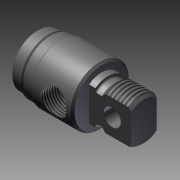
# Autodesk Inventor part: 04P0000_rear_head
Saved by Autodesk Inventor 2011 SP1 (Build 150282100, 282)
## iProperties
Created: 2015-01-23
Part Number: 04P0000_rear_head
Catalog Web Link: www.cadenas.de
Description: Rear Head-Original Line - Standard Air Cylinders
Vendor: BIMBA
Document SubType Name: Modeling
Designer: psAdmin
Manufacturer: BIMBA
Mass: 8.73981 g
Surface Area: 40.5299 cm^2
Volume: 8.73981 cm^3
Density: 1 g/cm^3
Category: PARTsolutions
Company: BIMBA
Title: 04P0000_rear_head
Author: Cadenas PARTsolutions
Comments: Original Line - Standard Air Cylinders
PSOL_IDENT_0: {$CADENAS_DATA\23d-libs\bimba\bimba\bimba_imperial\bimba_full_line\original_line_cylinders\standard_
PSOL_IDENT_1: air_cylinders\rear_head.prj},229 {VTYP=3D},{NB=04P0000_rear_head},{LINA=04P0000_rear_head},{NN=Rear
PSOL_IDENT_2: Head},{DATE=30.06.2014 06:34:23},{GEOMDATE=30.06.2014 06:34:00},{VERSION=},{LINEID=40},{LINESUBID=-1
PSOL_IDENT_3: },{WBVAR=MNT,ACTING,DER,Q,T1,T2,T3,T4,TRIM,Y,K,MB,CUSH,FBON}  {NB=04P0000_rear_head},{LINA=04P0000_r
PSOL_IDENT_4: ear_head},{KT=DUMMY},{PN=04P0000},{BORE=0.75000},{BOREPN=04},{MNT=P},{MNTALG='' , 'Front Nose' , 'P'
PSOL_IDENT_5: , 'Rear Pivot' , 'LS' , 'Built-in Valve LS' , 'DX' , 'Double End' , 'BR' , 'Rear Block' , 'BRT' , '
PSOL_IDENT_6: Rear Trunnion' , 'A' , 'Adjustable Stroke'},{ACTING=},{ACTINGALG= '' , 'Single Acting' , 'R' , 'Reve
PSOL_IDENT_7: rse/Double Acting'   },{DER=},{DERALG= '' , 'Standard' },{Q=},{T1=},{T2=},{T3=},{T4=},{TRIM=0},{Y=},
PSOL_IDENT_8: {K=},{KALG= '', 'without K', 'K', 'with K' },{MB=0},{A1=1.5940},{A1N=0.5310},{A1P=1.5940},{A1B=1.094
PSOL_IDENT_9: 0},{A1S=1.2190},{A2=0.219},{A2N=0.2190},{A3=0.0300},{D1=0.8625},{D1N=0.8050},{D1P=0.8625},{D1B=0.832
PSOL_IDENT_10: 5},{D2=0.7615},{C1=0.0300},{C2=0.0000},{NDM=0.4050},{TAB=NPT},{NDMDP=0.3020},{D3=0.3440},{A4=0.1880}
PSOL_IDENT_11: ,{A5=0.6200},{D4=0.0000},{A6=0.0000},{A7=0.7500},{A8=0.1250},{D5=0.8170},{D6=0.3120},{A9=0.8440},{ND
PSOL_IDENT_12: M2=0.6250},{TAB2=UNF},{C11=0.0300},{C22=0.0000},{C33=0.0227},{C44=0.0300},{A10=0.3725},{A11=0.0000},
PSOL_IDENT_13: {NDM3=0.4050},{NDM3N=0.4050},{NDM3B=0.4050},{TAB3=NPT},{TAB3N=NPT},{TAB3B=NPT},{A12=0.688},{A12N=0.6
PSOL_IDENT_14: 880},{A12B=0.6560},{A13=1.3120},{D7=0.2520},{D8=0.6225},{A14=0.0940},{A15=0.0855},{D9=0.5385},{R1=0.
PSOL_IDENT_15: 0350},{X1=0.0000},{X2=0.0000},{CX=0.0000},{CC=0.0000},{CON=1},{S1=1.0000},{DB=0.2500},{X1B=0.4380},{
PSOL_IDENT_16: X2B=0.0310},{A8B=0.1250},{A9B=0.8750},{MODEL=1},{NDM4=0.1900},{TAB4=UNF},{NDM4DP=0.2500},{BC=1.0000}
PSOL_IDENT_17: ,{B1=0.7150},{B2=0.5000},{B3=0.5000},{ON=0},{ON2=1},{G1=0.1250},{G2=0.5620},{G3=0.6250},{G4=0.6250},
PSOL_IDENT_18: {GD=0.2520},{G5=0.6250},{G6=0.3725},{RON=0},{H1=1.1175},{H2=0.8170},{H3=0.1250},{H4=0.0350},{H5=0.94
PSOL_IDENT_19: 20},{H6=0.5620},{F=0.4380},{PNUT=1.0630},{CUSH=0},{CC11=0.238},{CC111=0.2380},{CC22=0.2750},{CC33=0.
PSOL_IDENT_20: 1950},{CC44=0.3700},{CC55=0.5350},{CD1=0.1900},{CD2=0.1500},{CD3=0.0725},{CNDM3=0.1380},{CTAB3=UNF},
PSOL_IDENT_21: {OLEN=1.3120},{OD=0.3455},{STDIS=0.1560},{STDIS1=0.1560},{BUSHCON=D-3543},{BUSHL=0.3700},{FBON=0},{L
PSOL_IDENT_22: CD=0.0000}
SUPPLIER: BIMBA
ARTICLENO: 04P0000_rear_head
BOMINFO: 04P0000_rear_head
CREATOR: CADENAS GmbH
Autodesk Inventor part; units mm, degrees
ref_plane "YZ Plane" through (0, 0, 0) normal (1, 0, 0) x (0, 1, 0)
ref_plane "XZ Plane" through (0, 0, 0) normal (0, 1, 0) x (-1, 0, 0)
ref_plane "XY Plane" through (0, 0, 0) normal (0, 0, 1) x (1, 0, 0)
sketch "Sketch_8" plane through (0, 0, 0) normal (0, 0, 1) x (1, 0, 0)
  line L0 (24.6126, 0) -> (0, 0)
  line L1 (0, 0) -> (0, 8.9091)
  line L2 (0, 8.9091) -> (0.762, 9.671)
  line L3 (0.762, 9.671) -> (4.0386, 9.671)
  line L4 (4.0386, 9.671) -> (4.8006, 8.9091)
  line L5 (4.8006, 8.9091) -> (5.5626, 8.9091)
  line L6 (5.5626, 8.9091) -> (5.5626, 10.3759)
  line L7 (5.5626, 10.3759) -> (8.7363, 10.3759)
  line L8 (8.7363, 10.3759) -> (9.3142, 10.9537)
  line L9 (9.3142, 10.9537) -> (23.8506, 10.9537)
  line L10 (23.8506, 10.9537) -> (24.6126, 10.1918)
  line L11 (24.6126, 10.1918) -> (24.6126, 0)
  line L12 (24.6126, 0) -> (0, 0)
  constraints: 26 end point
revolve "Revolution1" add sketch "Sketch_8" angle 360 about axis through (24.6126, 0, 0) along (1, 0, 0)
sketch "Sketch_15" plane through (0, 0, 0) normal (0, 0, 1) x (1, 0, 0)
  line L0 (40.4876, 0) -> (24.6126, 0)
  line L1 (24.6126, 0) -> (24.6126, 7.9057)
  line L2 (24.6126, 7.9057) -> (27.0002, 7.9057)
  line L3 (27.0002, 7.9057) -> (27.0002, 7.7279)
  arc A0 (27.0002, 7.7279) -> (27.8892, 6.839) centre (27.8892, 7.7279) ccw
  line L4 (27.8892, 6.839) -> (29.1719, 6.839)
  arc A1 (29.1719, 6.839) -> (29.7706, 7.0708) centre (29.1719, 7.7279) ccw
  line L5 (29.7706, 7.0708) -> (29.8005, 7.098)
  line L6 (29.8005, 7.098) -> (30.64, 7.9375)
  line L7 (30.64, 7.9375) -> (39.6481, 7.9375)
  line L8 (39.6481, 7.9375) -> (40.4876, 7.098)
  line L9 (40.4876, 7.098) -> (40.4876, 0)
  line L10 (40.4876, 0) -> (24.6126, 0)
  constraints: 22 end point, 4 point on circle, 2 centre point
revolve "Revolution2" add sketch "Sketch_15" angle 360 about axis through (40.4876, 0, 0) along (1, 0, 0)
thread "Thread1" size "5/8-18 UNF" class "2A" standard "ANSI Unified Screw Threads" full length
sketch "Sketch_9" plane through (40.4876, 0, 0) normal (1, 0, 0) x (0, 0, -1)
  line L0 (-21.9075, -43.815) -> (21.9075, -43.815)
  line L1 (21.9075, -43.815) -> (21.9075, 43.815)
  line L2 (21.9075, 43.815) -> (-21.9075, 43.815)
  line L3 (-21.9075, 43.815) -> (-21.9075, -43.815)
  line L4 (-4.7307, -21.9075) -> (4.7307, -21.9075)
  line L5 (4.7307, -21.9075) -> (4.7307, 21.9075)
  line L6 (4.7307, 21.9075) -> (-4.7307, 21.9075)
  line L7 (-4.7307, 21.9075) -> (-4.7307, -21.9075)
  constraints: 16 end point
extrude "Extrusion1" cut sketch "Sketch_9" against normal blind 15.875
sketch "Sketch4" plane through (0, 0, 0) normal (-1, 0, 0) x (0, 0, 1)
  point P0 (0, 0)
hole "Hole1" at (0, 0, 0) direction (1, 0, 0) diameter 7.9248 depth 23.5814 tip angle 120
sketch "Sketch_68" plane through (0, 0, 0) normal (0, 0.9998477, 0.0174524) x (1, 0, 0)
  line L0 (17.4752, -10.9537) -> (17.4752, 0)
  line L1 (17.4752, 0) -> (22.0752, 0)
  line L2 (22.0752, 0) -> (22.0752, -3.2829)
  line L3 (22.0752, -3.2829) -> (22.3147, -10.9537)
  line L4 (22.3147, -10.9537) -> (17.4752, -10.9537)
  line L5 (17.4752, -10.9537) -> (17.4752, 0)
  constraints: 12 end point
revolve "Revolution3" cut sketch "Sketch_68" angle 360 about axis through (17.4752, -0.1912, 10.9521) along (0, -0.0174524, 0.9998477)
thread "Thread2" size "1/8" designation "1/8 - 27 NPT" standard "NPT" full length
sketch "Sketch_24" plane through (0, 0, 0) normal (0, 0, 1) x (1, 0, 0)
  line L0 (5.5626, 0) -> (4.8006, 0)
  line L1 (4.4955, 10.2917) -> (5.4401, 9.3472)
  arc A0 (5.4401, 9.1676) -> (5.4401, 9.3472) centre (5.3503, 9.2574) ccw
  line L2 (5.4401, 9.1676) -> (5.1816, 8.9091)
  line L3 (5.1816, 8.9091) -> (4.8006, 8.9091)
  line L4 (4.8006, 8.9091) -> (4.8006, 8.655)
  line L5 (4.8006, 8.655) -> (5.5626, 8.655)
  line L6 (5.5626, 8.655) -> (5.5626, 9.512)
  line L7 (5.5626, 9.512) -> (4.6987, 10.3759)
  line L8 (4.6987, 10.3759) -> (4.4955, 10.3759)
  line L9 (4.4955, 10.3759) -> (4.4955, 10.2917)
  constraints: 20 end point, 2 point on circle, 1 centre point
revolve "Revolution4" add sketch "Sketch_24" angle 360 about axis through (5.5626, 0, 0) along (1, 0, 0)
sketch "Sketch_43" plane through (0, 0, 0) normal (0, 0, 1) x (1, 0, 0)
  circle A0 centre (33.3248, 0) radius 3.2004
  constraints: 1 centre point
extrude "Extrusion2" cut sketch "Sketch_43" along normal mid plane 14.1922
ref_plane "1_XY" through (27.0002, 0, 0) normal (1, 0, 0) x (0, 0, -1)
ref_plane "1_YZ" through (27.0002, 0, 0) normal (0, 0, -1) x (0, 1, 0)
ref_plane "1_ZX" through (27.0002, 0, 0) normal (0, 1, 0) x (1, 0, 0)
ref_plane "c1_XY" through (24.6126, 7.9057, 0) normal (0, 0, 1) x (1, 0, 0)
ref_plane "c1_YZ" through (24.6126, 7.9057, 0) normal (1, 0, 0) x (0, 1, 0)
ref_plane "c1_ZX" through (24.6126, 7.9057, 0) normal (0, 1, 0) x (0, 0, 1)
ref_plane "c2_XY" through (24.6126, -7.9057, 0) normal (0, 0, 1) x (1, 0, 0)
ref_plane "c2_YZ" through (24.6126, -7.9057, 0) normal (1, 0, 0) x (0, 1, 0)
ref_plane "c2_ZX" through (24.6126, -7.9057, 0) normal (0, 1, 0) x (0, 0, 1)
ref_plane "cc1_XY" through (24.6126, 0, 0) normal (0, 0, 1) x (1, 0, 0)
ref_plane "cc1_YZ" through (24.6126, 0, 0) normal (1, 0, 0) x (0, 1, 0)
ref_plane "cc1_ZX" through (24.6126, 0, 0) normal (0, 1, 0) x (0, 0, 1)
ref_plane "cc2_XY" through (27.0002, 0, 0) normal (0, 0, 1) x (1, 0, 0)
ref_plane "cc2_YZ" through (27.0002, 0, 0) normal (1, 0, 0) x (0, 1, 0)
ref_plane "cc2_ZX" through (27.0002, 0, 0) normal (0, 1, 0) x (0, 0, 1)
ref_plane "lovra1_XY" through (35.7124, 0, 0) normal (1, 0, 0) x (0, 0, -1)
ref_plane "lovra1_YZ" through (35.7124, 0, 0) normal (0, 0, -1) x (0, 1, 0)
ref_plane "lovra1_ZX" through (35.7124, 0, 0) normal (0, 1, 0) x (1, 0, 0)
ref_plane "lovra2_XY" through (35.7124, 7.874, 0) normal (1, 0, 0) x (0, 0, -1)
ref_plane "lovra2_YZ" through (35.7124, 7.874, 0) normal (0, 0, -1) x (0, 1, 0)
ref_plane "lovra2_ZX" through (35.7124, 7.874, 0) normal (0, 1, 0) x (1, 0, 0)
ref_plane "lovra21_XY" through (0, 0, 5.2705) normal (1, 0, 0) x (0, 0, -1)
ref_plane "lovra21_YZ" through (0, 0, 5.2705) normal (0, 0, -1) x (0, 1, 0)
ref_plane "lovra21_ZX" through (0, 0, 5.2705) normal (0, 1, 0) x (1, 0, 0)
ref_plane "lovra22_XY" through (0, 0, -5.2705) normal (1, 0, 0) x (0, 0, -1)
ref_plane "lovra22_YZ" through (0, 0, -5.2705) normal (0, 0, -1) x (0, 1, 0)
ref_plane "lovra22_ZX" through (0, 0, -5.2705) normal (0, 1, 0) x (1, 0, 0)
ref_plane "lovra3_XY" through (35.7124, -7.874, 0) normal (1, 0, 0) x (0, 0, -1)
ref_plane "lovra3_YZ" through (35.7124, -7.874, 0) normal (0, 0, -1) x (0, 1, 0)
ref_plane "lovra3_ZX" through (35.7124, -7.874, 0) normal (0, 1, 0) x (1, 0, 0)
ref_plane "olen_XY" through (33.3248, 0, 0) normal (1, 0, 0) x (0, 0, -1)
ref_plane "olen_YZ" through (33.3248, 0, 0) normal (0, 0, -1) x (0, 1, 0)
ref_plane "olen_ZX" through (33.3248, 0, 0) normal (0, 1, 0) x (1, 0, 0)
ref_plane "p1_XY" through (40.4876, 0, 4.7307) normal (1, 0, 0) x (0, 0, -1)
ref_plane "p1_YZ" through (40.4876, 0, 4.7307) normal (0, 0, -1) x (0, 1, 0)
ref_plane "p1_ZX" through (40.4876, 0, 4.7307) normal (0, 1, 0) x (1, 0, 0)
ref_plane "p2_XY" through (40.4876, 0, -4.7307) normal (1, 0, 0) x (0, 0, -1)
ref_plane "p2_YZ" through (40.4876, 0, -4.7307) normal (0, 0, -1) x (0, 1, 0)
ref_plane "p2_ZX" through (40.4876, 0, -4.7307) normal (0, 1, 0) x (1, 0, 0)
ref_plane "port_XY" through (17.4752, 0, 0) normal (0, 0, 1) x (1, 0, 0)
ref_plane "port_YZ" through (17.4752, 0, 0) normal (1, 0, 0) x (0, 1, 0)
ref_plane "port_ZX" through (17.4752, 0, 0) normal (0, 1, 0) x (0, 0, 1)
ref_plane "port2_XY" through (40.4876, 0, 0) normal (1, 0, 0) x (0, 0, -1)
ref_plane "port2_YZ" through (40.4876, 0, 0) normal (0, 0, -1) x (0, 1, 0)
ref_plane "port2_ZX" through (40.4876, 0, 0) normal (0, 1, 0) x (1, 0, 0)
ref_plane "thd1_XY" through (40.4876, 0, 7.9375) normal (1, 0, 0) x (0, 0, -1)
ref_plane "thd1_YZ" through (40.4876, 0, 7.9375) normal (0, 0, -1) x (0, 1, 0)
ref_plane "thd1_ZX" through (40.4876, 0, 7.9375) normal (0, 1, 0) x (1, 0, 0)
ref_plane "thd2_XY" through (40.4876, 0, -7.9375) normal (1, 0, 0) x (0, 0, -1)
ref_plane "thd2_YZ" through (40.4876, 0, -7.9375) normal (0, 0, -1) x (0, 1, 0)
ref_plane "thd2_ZX" through (40.4876, 0, -7.9375) normal (0, 1, 0) x (1, 0, 0)
ref_plane "to_mounting_bracket_XY" through (24.6126, 0, 0) normal (1, 0, 0) x (0, 0, -1)
ref_plane "to_mounting_bracket_YZ" through (24.6126, 0, 0) normal (0, 0, -1) x (0, 1, 0)
ref_plane "to_mounting_bracket_ZX" through (24.6126, 0, 0) normal (0, 1, 0) x (1, 0, 0)
ref_plane "to_nut_XY" through (27.0002, 0, 0) normal (1, 0, 0) x (0, 0, -1)
ref_plane "to_nut_YZ" through (27.0002, 0, 0) normal (0, 0, -1) x (0, 1, 0)
ref_plane "to_nut_ZX" through (27.0002, 0, 0) normal (0, 1, 0) x (1, 0, 0)
ref_plane "to_pin_XY" through (33.3248, 0, 0) normal (0, 0, 1) x (1, 0, 0)
ref_plane "to_pin_YZ" through (33.3248, 0, 0) normal (1, 0, 0) x (0, 1, 0)
ref_plane "to_pin_ZX" through (33.3248, 0, 0) normal (0, 1, 0) x (0, 0, 1)
ref_plane "to_screw_XY" through (17.4752, 2.032, -6.0452) normal (0, 1, 0) x (1, 0, 0)
ref_plane "to_screw_YZ" through (17.4752, 2.032, -6.0452) normal (1, 0, 0) x (0, 0, -1)
ref_plane "to_screw_ZX" through (17.4752, 2.032, -6.0452) normal (0, 0, -1) x (0, 1, 0)
ref_plane "to_tube_XY" through (4.8006, 0, 0) normal (1, 0, 0) x (0, 0, -1)
ref_plane "to_tube_YZ" through (4.8006, 0, 0) normal (0, 0, -1) x (0, 1, 0)
ref_plane "to_tube_ZX" through (4.8006, 0, 0) normal (0, 1, 0) x (1, 0, 0)
body "Solid1"
